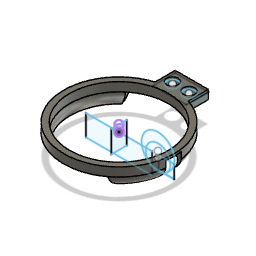
Watch_Holder_Top_curvededge v7 (Autodesk Fusion 360 design; units mm, degrees)
Autodesk Fusion 360 part; units mm, degrees
note: some values were not read from the file. Set by a fixed rule: which sketch regions a step uses.
sketch "Sketch1" plane through (0, 0, 0) normal (0, 1, 0) x (1, 0, 0)
  circle A0 centre (0, 0) radius 22.375
  circle A1 centre (0, 0) radius 25
  dimension "d1" = 44.75
  dimension "d2" = 50
  constraint coincident A0.centre A1.centre
  constraint concentric A0 A1
  measures "d1" diameter of A0
  measures "d2" diameter of A1
sketch "Sketch2" plane through (0, 0, 0) normal (0, 0, 1) x (1, 0, 0)
extrude "Extrude1" add sketch "Sketch1" along normal blind 3
sketch "Sketch3" plane through (0, 0, 0) normal (0, 0, 1) x (1, 0, 0)
  line L0 (18, 0) -> (18, -6)
  line L1 (25, 0) -> (25, -6)
  line L2 (18, -6) -> (25, -6)
  line L3 (18, 0) -> (25, 0)
  line L4 (18, -6) -> (25, -6)
  circle A0 centre (17.7502, -1.1354) radius 5.5639
  circle A1 centre (17.685, 1.409) radius 7.4494
  dimension "d9" = 18
  dimension "d10" = 25
  dimension "d11" = 6
  dimension "d12" = 6
  constraint vertical L0
  constraint vertical L1
  constraint perpendicular L1 L2
  constraint coincident L1.start A1
  measures "d9" horizontal distance of L0.start origin
  measures "d10" horizontal distance of origin L1.start
  measures "d11" distance of L0.start L0.end
  measures "d12" distance of L1.start L1.end
sketch "Sketch4" plane through (0, 0, 0) normal (0, 0, 1) x (1, 0, 0)
sketch "Sketch5" plane through (0, 0, 0) normal (0, 0, 1) x (1, 0, 0)
  line L0 (-15, -0.0108) -> (15, -0.0108)
  line L1 (15, -0.0108) -> (15, -9.5655)
  line L2 (15, -9.5655) -> (-15, -9.5655)
  line L3 (-15, -9.5655) -> (-15, -0.0108)
  dimension "d14" = 30
  dimension "d15" = 15
  constraint horizontal L0
  constraint vertical L1
  constraint horizontal L2
  constraint vertical L3
  measures "d14" distance of L0.start L0.end
  measures "d15" horizontal distance of origin L0.start
sketch "Sketch6" plane through (0, 3, 0) normal (0, 1, 0) x (-1, 0, 0)
  circle A0 centre (0, 0) radius 22.375
  circle A1 centre (0, 0) radius 25
sketch "Sketch7" plane through (0, 0, 0) normal (1, 0, 0) x (0, 0, -1)
  line L0 (-3.5, 2.9971) -> (3.5, 2.9971)
  line L1 (3.5, 2.9971) -> (3.5, -7)
  line L2 (3.5, -7) -> (-3.5, -7)
  line L3 (-3.5, -7) -> (-3.5, 2.9971)
  point P0 (0, 1.409)
  dimension "d20" = 7
  dimension "d26" = 3.5
  constraint horizontal L0
  constraint vertical L1
  constraint horizontal L2
  constraint vertical L3
  measures "d20" distance of L0.start L0.end
  measures "d26" horizontal distance of L0.end P0
sketch "Sketch8" plane through (0, 0, 0) normal (0, 0, 1) x (1, 0, 0)
sketch "Sketch9" plane through (0, 3, 0) normal (0, 1, 0) x (-1, 0, 0)
extrude "Extrude4" cut sketch "Sketch7" along normal blind 25
extrude "Extrude5" cut sketch "Sketch5" along normal blind 32 and the other way blind 36
sketch "Sketch10" plane through (0, 3, 0) normal (0, 1, 0) x (-1, 0, 0)
  line L0 (7.5, -33) -> (-7.5, -33)
  line L1 (-7.5, -33) -> (-7.5, -23)
  line L2 (-7.5, -23) -> (7.5, -23)
  line L3 (7.5, -23) -> (7.5, -33)
  circle A0 centre (3.75, -28) radius 2.6
  circle A1 centre (-3.75, -28) radius 2.6
  dimension "d33" = 15
  dimension "d34" = 7.5
  dimension "d35" = 5.2
  dimension "d36" = 5.2
  dimension "d37" = 10
  dimension "d38" = 23
  dimension "d39" = 3.75
  dimension "d40" = 3.75
  constraint horizontal L0
  constraint vertical L1
  constraint horizontal L2
  constraint vertical L3
  measures "d33" distance of L0.start L0.end
  measures "d34" horizontal distance of L1.end origin
  measures "d35" diameter of A1
  measures "d36" diameter of A0
  measures "d37" distance of L0.end L1.end
  measures "d38" vertical distance of L2.end origin
  measures "d39" horizontal distance of A0.centre origin
  measures "d40" horizontal distance of A1.centre origin
revolve "Revolve4" add sketch "Sketch3" angle 360 about axis through (0, 1.75, 0) along (0, 1, 0) contours L3 A0 A1 picked at (24.3244, -0.4805)
extrude "Extrude9" cut sketch "Sketch5" along normal blind 42 and the other way blind 47
extrude "Extrude10" cut sketch "Sketch7" along normal blind 53
sketch "Sketch11" plane through (0, 0, 0) normal (0, 0, 1) x (1, 0, 0)
sketch "Sketch12" plane through (0, 0, 0) normal (0, 1, 0) x (1, 0, 0)
extrude "Extrude11" add sketch "Sketch10" against normal blind 3
extrude "Extrude12" add 1 faces at (1.0571, 3, -32.1783) along direction (0, 1, 0) blind 1
sketch "Sketch13" plane through (0, 0, 0) normal (0, 0, 1) x (1, 0, 0)
sketch "Sketch14" plane through (0, 0, 0) normal (1, 0, 0) x (0, 0, -1)
sketch "Sketch15" plane through (7.5, 0, 0) normal (1, 0, 0) x (0, 0, -1)
  line L0 (23.8485, 4) -> (23.8485, 0)
  line L1 (23.8485, 0) -> (33, 0)
  line L2 (33, 0) -> (33, 4)
  line L3 (33, 4) -> (23.8485, 4)
sketch "Sketch16" plane through (0, 0, 0) normal (1, 0, 0) x (0, 0, -1)
equation "d10 = ( 50 / 2 ) * 1 mm"
equation "d39 = ( 7.5 / 2 ) * 1 mm"
